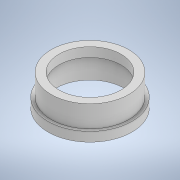
# Autodesk Inventor part: bearing_adapter_sleeve
Saved by Autodesk Inventor 2020 (Build 240168000, 168)
## iProperties
Created: 2020-03-12
Part Number: bearing_adapter_sleeve
Material: Generic
Document SubType Name: Modeling
Designer: erwin
Density: 1 g/cm^3
Appearance: Default
Author: erwin
Autodesk Inventor part; units mm, degrees
ref_plane "YZ Plane" through (0, 0, 0) normal (1, 0, 0) x (0, 1, 0)
ref_plane "XZ Plane" through (0, 0, 0) normal (0, 1, 0) x (-1, 0, 0)
ref_plane "XY Plane" through (0, 0, 0) normal (0, 0, 1) x (1, 0, 0)
sketch "Sketch1" plane through (0, 0, 0) normal (0, 1, 0) x (-1, 0, 0)
  circle A0 centre (0, 0) radius 12.5
  circle A1 centre (0, 0) radius 11
  dimension "d0" = 25
  dimension "d1" = 22
  constraints: 2 centre point, 2 coincident
  measures "d0" diameter of A0
  measures "d1" diameter of A1
extrude "Extrusion1" add sketch "Sketch1" along normal blind 10
sketch "Sketch2" plane through (0, 10, 0) normal (0, 1, 0) x (1, 0, 0)
  circle A0 centre (0, 0) radius 12.5 projected
  circle A1 centre (0, 0) radius 11 projected
  circle A2 centre (0, 0) radius 10
  dimension "d4" = 1
  constraints: 1 centre point
  measures "d4" radial gap between concentric circles of A1 A2
extrude "Extrusion2" add sketch "Sketch2" against normal blind 3 contours A1
sketch "Sketch3" plane through (0, 0, 0) normal (0, -1, 0) x (1, 0, 0)
  circle A0 centre (0, 0) radius 12.5 projected
  circle A1 centre (0, 0) radius 11 projected
  circle A2 centre (0, 0) radius 13.5
  dimension "d7" = 1
  constraints: 1 centre point
  measures "d7" radial gap between concentric circles of A0 A2
extrude "Extrusion3" add sketch "Sketch3" against normal blind 3 contours A2
body "Solid1"
